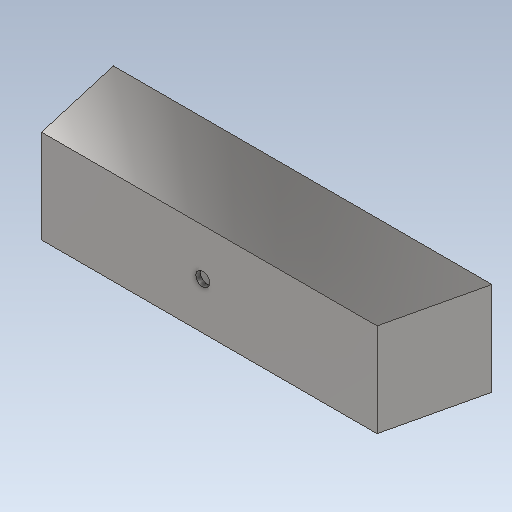
# Autodesk Inventor part: v chasis
Saved by Autodesk Inventor 2020 (Build 240168000, 168)
## iProperties
Created: 2019-07-22
Part Number: v chasis
Material: Steel, Mild
Document SubType Name: Modeling
Designer: BARLY
Density: 7.85 g/cm^3
Appearance: Semi-Polished
Mass: 6344.39 g
Surface Area: 3239.58 cm^2
Volume: 808.203 cm^3
Author: BARLY
Autodesk Inventor part; units mm, degrees
ref_plane "YZ Plane" through (0, 0, 0) normal (1, 0, 0) x (0, 1, 0)
ref_plane "XZ Plane" through (0, 0, 0) normal (0, 1, 0) x (-1, 0, 0)
ref_plane "XY Plane" through (0, 0, 0) normal (0, 0, 1) x (1, 0, 0)
sketch "Sketch1" plane through (0, 0, 0) normal (0, 1, 0) x (-1, 0, 0)
  line L0 (0, 0) -> (-359.4604, 0)
  line L1 (-173.205, -100) -> (23.0868, -100)
  line L2 (23.0868, -100) -> (-382.5472, -100)
  line L3 (-382.5472, -100) -> (-359.4604, 0)
  line L4 (23.0868, -100) -> (0, 0)
  dimension "d16" = 103
  dimension "d17" = 100
  dimension "d18" = 405.634
  dimension "d19" = 103
  constraints: 10 end point, 2 horizontal
  measures "d16" angle of L0 L3
  measures "d17" distance between parallel lines of L0 L1
  measures "d18" distance of L1.end L2.end
  measures "d19" angle of L4 L0
extrude "Extrusion1" add sketch "Sketch1" along normal blind 5
sketch "Sketch2" plane through (0, 5, 0) normal (0, 1, 0) x (1, 0, 0)
  line L0 (-23.0868, 100) -> (0, 0) projected
  line L1 (0, 0) -> (-23.0868, 100)
  line L2 (382.5472, 100) -> (-23.0868, 100) projected
  line L3 (-23.0868, 100) -> (382.5472, 100)
  line L4 (359.4604, 0) -> (382.5472, 100) projected
  line L5 (382.5472, 100) -> (359.4604, 0)
  line L6 (359.4604, 0) -> (0, 0)
  line L7 (3.9772, 5) -> (-16.801, 95)
  line L8 (-16.801, 95) -> (376.2613, 95)
  line L9 (376.2613, 95) -> (355.4832, 5)
  line L10 (355.4832, 5) -> (3.9772, 5)
  dimension "d6" = 5
  constraints: 16 end point, 3 collinear, 2 parallel, 3 other
  measures "d6" distance between parallel lines of L6 L10
extrude "Extrusion2" add sketch "Sketch2" along normal blind 90
sketch "Sketch3" plane through (0, 0, 0) normal (0, 0, 1) x (1, 0, 0)
  line L0 (0, 0) -> (0, 50)
  line L1 (0, 0) -> (0, 95) projected
  line L2 (0, 50) -> (345.363, 50)
  circle A0 centre (172.6815, 50) radius 7.5
  dimension "d9" = 50
  dimension "d10" = 15
  constraints: 4 end point, 1 centre point, 1 midpoint, 1 perpendicular, 1 point on line
  measures "d9" distance of L0.start L0.end
  measures "d10" diameter of A0
extrude "Extrusion3" cut sketch "Sketch3" against normal blind 455
sketch "Sketch4" plane through (0, 95, 0) normal (0, 1, 0) x (1, 0, 0)
  line L0 (-23.0868, 100) -> (0, 0) projected
  line L1 (0, 0) -> (-23.0868, 100)
  line L2 (359.4604, 0) -> (382.5472, 100) projected
  line L3 (-23.0868, 100) -> (382.5472, 100)
  line L4 (382.5472, 100) -> (359.4604, 0)
  line L5 (359.4604, 0) -> (0, 0)
  line L6 (355.4832, 5) -> (3.9772, 5) projected
  constraints: 8 end point, 2 collinear, 1 horizontal, 1 parallel
extrude "Extrusion4" add sketch "Sketch4" along normal blind 5
body "Solid1"
